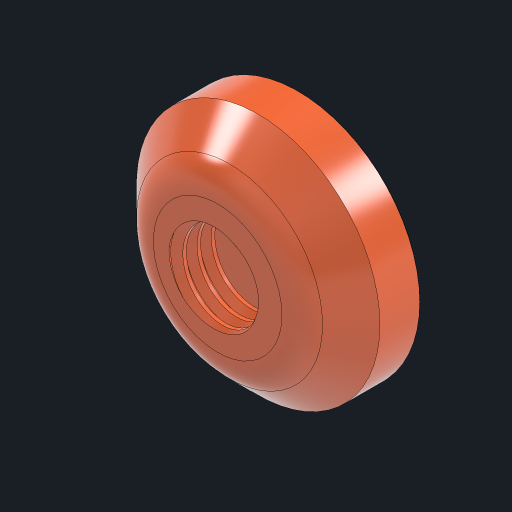
# Autodesk Inventor part: SKÅDIS Pegboard Clamp3
Saved by Autodesk Inventor 2024 (Build 280153000, 153)
## iProperties
Created: 2024-02-08
Part Number: SKÅDIS Pegboard Clamp3
Material: 일반
Document SubType Name: Modeling
Designer: KBU
Density: 1 g/cm^3
Appearance: 기본값
Author: KBU
Autodesk Inventor part; units mm, degrees
ref_plane "YZ Plane" through (0, 0, 0) normal (1, 0, 0) x (0, 1, 0)
ref_plane "XZ Plane" through (0, 0, 0) normal (0, 1, 0) x (-1, 0, 0)
ref_plane "XY Plane" through (0, 0, 0) normal (0, 0, 1) x (1, 0, 0)
sketch "스케치1" plane through (0, 0, 0) normal (0, 0, 1) x (1, 0, 0)
  circle A0 centre (0, 0) radius 15
  dimension "d0" = 30
  constraints: 1 centre point, 1 coincident
  measures "d0" diameter of A0
extrude "돌출1" add sketch "스케치1" along normal blind 10
sketch "스케치2" plane through (0, 0, 10) normal (0, 0, 1) x (1, 0, 0)
  circle A0 centre (0, 0) radius 15 projected
  circle A1 centre (0, 0) radius 6
  dimension "d3" = 12
  constraints: 1 centre point, 1 coincident
  measures "d3" diameter of A1
extrude "돌출2" cut sketch "스케치2" against normal blind 5 contours A1
sketch "스케치3" plane through (0, 0, 0) normal (0, 1, 0) x (-1, 0, 0)
  line L0 (0, 14.7828) -> (0, -0.3164)
  line L1 (6.1894, 11.6406) -> (6.1894, 9.8906)
  line L2 (6.1894, 9.8906) -> (4.6739, 10.7656)
  line L3 (4.6739, 10.7656) -> (6.1894, 11.6406)
  line L4 (6, 11.5312) -> (6, 10) construction
  line L5 (5.053, 10.9845) -> (5.053, 10.5468)
  line L6 (-6, 10) -> (6, 10) projected
  point P0 (0, 0)
  point P1 (5.053, 10.7656)
  dimension "d6" = 60
  dimension "d7" = 60
  dimension "d8" = 1.75
  dimension "d9" = 12
  dimension "d10" = 10.106
  dimension "d11" = 1.5155
  dimension "d12" = 0.1894
  dimension "d13" = 0.947
  dimension "d14" = 0
  constraints: 12 end point, 5 vertical, 4 point on line, 1 midpoint
  measures "d6" angle of L1 L3
  measures "d7" angle of L2 L1
  measures "d8" distance of L1.start L1.end
  measures "d9" diameter of L4 L0
  measures "d10" diameter of point (5.053, 10.766) L0
  measures "d11" distance from line of L2.end L1
  measures "d12" distance between parallel lines of L4 L1
  measures "d13" distance from line of L4 point (5.053, 10.766)
  measures "d14" distance from line of L6 L4.end
coil "코일1" sketch "스케치3" operation add axis through (0, 0, 14.7828) along (0, 0, -1) pitch 1.75 turns 4 hand right contours L1 L2 L5 L3
sketch "스케치4" plane through (0, 0, 10) normal (0, 0, 1) x (1, 0, 0)
  line L0 (-6, 0) -> (-6.1894, 0) projected
  arc A0 (-5.7183, -2.3686) -> (-6.1894, 0) centre (0, 0) ccw projected
  spline S0 degree 7 poles (-5.7183, -2.3686) (-5.5809, -2.6388) (-5.428, -2.9011) (-5.2601, -3.1544) (-5.0778, -3.3976) (-4.8817, -3.6296) (-4.6727, -3.8495) (-4.4222, -4.0837) (-4.3928, -4.1108) (-4.3632, -4.1376) (-4.3333, -4.1642) (-4.3033, -4.1906) (-4.273, -4.2168) (-4.2426, -4.2427) knots 0 0 0 0 0 0 0 0 0.883338 0.883338 0.883338 0.883338 0.883338 0.883338 1 1 1 1 1 1 1 1 projected
  arc A1 (-6, 0) -> (-4.2426, -4.2426) centre (0, 0) ccw projected
  constraints: 1 other
extrude "돌출3" cut sketch "스케치4" along normal blind 5
sketch "스케치5" plane through (0, 0, 5) normal (0, 0, 1) x (1, 0, 0)
  arc A0 (4.4236, 2.4423) -> (-2.4462, 4.4214) centre (0, 0) ccw projected
  circle A1 centre (0, 0) radius 7.5
  dimension "d25" = 15
  constraints: 1 centre point, 1 coincident
  measures "d25" diameter of A1
extrude "돌출4" cut sketch "스케치5" against normal blind 1
chamfer "모따기2" distance 5 angle 45 1 edges at (-15, 0, 10)
fillet "모깎기1" radius 5 1 edges at (-10, 0, 10)
chamfer "모따기3" distance 0.1 angle 45 1 edges at (-15, 0, 0)
equation "\"d12\" = 0.125 * d11"
